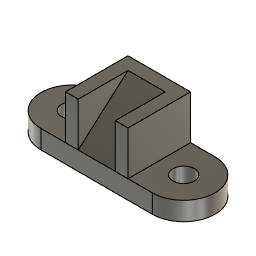
A2 (Autodesk Fusion 360 design; units mm, degrees)
Autodesk Fusion 360 part; units mm, degrees
sketch "Sketch1" plane through (0, 0, 0) normal (0, 0, 1) x (1, 0, 0)
  line L0 (57, 32) -> (-57, 32)
  line L1 (-57, -32) -> (57, -32)
  circle A0 centre (57, 0) radius 11
  circle A1 centre (-57, 0) radius 11
  arc A2 (-57, 32) -> (-57, -32) centre (-57, 0) ccw
  arc A3 (57, -32) -> (57, 32) centre (57, 0) ccw
  dimension "d1" = 114
  dimension "d2" = 64
  dimension "d3" = 22
  dimension "d4" = 22
  constraint horizontal L0
  constraint parallel L0 L1
  constraint concentric A0 A3
  constraint concentric A1 A2
  measures "d1" distance of L1.start L1.end
  measures "d2" distance of L0.end L1.start
  measures "d3" diameter of A0
  measures "d4" diameter of A1
extrude "Extrude1" add sketch "Sketch1" along normal blind 19 makes body 1
sketch "Sketch2" plane through (0, 0, 0) normal (1, 0, 0) x (0, 1, 0)
  line L0 (-32, 19) -> (19, 19)
  line L1 (19, 19) -> (19, 64)
  line L2 (19, 64) -> (-32, 19)
  dimension "d7" = 51
  dimension "d8" = 45
  constraint horizontal L0
  constraint perpendicular L0 L1
  measures "d7" distance of L0.start L0.end
  measures "d8" distance of L0.end L1.end
extrude "Extrude2" add sketch "Sketch2" along normal mid plane 38 bodies 1
sketch "Sketch3" plane through (0, 0, 19) normal (0, 0, 1) x (-1, 0, 0)
  line L0 (-19, -19) -> (-19, 32)
  line L1 (-19, 32) -> (-57, 32)
  arc A0 (-57, 32) -> (-57, -32) centre (-57, 0) ccw
  line L2 (-57, -32) -> (57, -32)
  arc A1 (57, -32) -> (57, 32) centre (57, 0) ccw
  line L3 (57, 32) -> (19, 32)
  line L4 (19, 32) -> (19, -19)
  line L5 (19, -19) -> (-19, -19)
  circle A2 centre (57, 0) radius 11
  circle A3 centre (-57, 0) radius 11
  line L6 (32, -32) -> (32, 32)
  line L7 (-32, -32) -> (-32, 32)
  dimension "d11" = 64
  dimension "d12" = 64
  dimension "d13" = 64
  dimension "d14" = 13
  constraint perpendicular L2 L6
  constraint coincident L2 L6.start
  constraint coincident L2 L7.start
  measures "d11" distance of L6.start L6.end
  measures "d12" distance of L7.end L7.start
  measures "d13" distance of L6 L7
  measures "d14" distance of L4 L6
extrude "Extrude3" add sketch "Sketch3" along normal blind 45 separate body contours L0 L1 L2 L3 L4 L5 L6 L7 makes body 2
combine "Combine1" operation add target body 2 tool bodies 1
equation "d8 = 64 mm - 19 mm"
equation "d15 = 64 mm - 19 mm"
